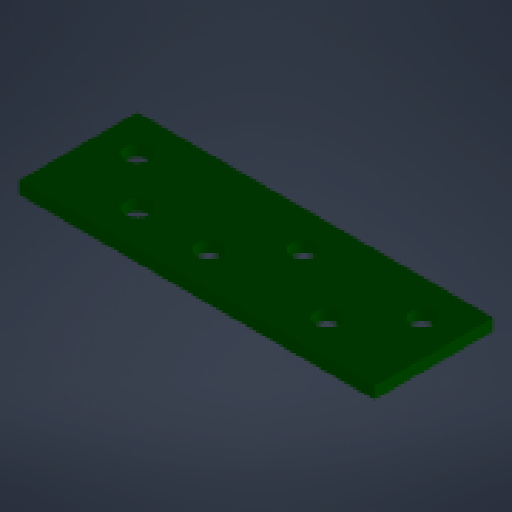
# Autodesk Inventor part: upper_plate
Saved by Autodesk Inventor 2024 (Build 280153000, 153)
## iProperties
Created: 2023-04-16
Part Number: upper_plate
Material: Типовые
Document SubType Name: Modeling
Designer: user
Density: 1 g/cm^3
Appearance: По умолчанию
Author: user
Autodesk Inventor part; units mm, degrees
ref_plane "YZ Plane" through (0, 0, 0) normal (1, 0, 0) x (0, 1, 0)
ref_plane "XZ Plane" through (0, 0, 0) normal (0, 1, 0) x (-1, 0, 0)
ref_plane "XY Plane" through (0, 0, 0) normal (0, 0, 1) x (1, 0, 0)
sketch "Эскиз1" plane through (0, 0, 0) normal (0, 0, 1) x (1, 0, 0)
  line L0 (-10, 0) -> (10, 0) projected
  line L1 (-10, 0) -> (-60, 0) projected
  line L2 (10, -20) -> (60, -20) projected
  circle A0 centre (-16, -14) radius 2 projected
  circle A1 centre (-24, -6) radius 2 projected
  circle A2 centre (-4, -14) radius 2 projected
  circle A3 centre (4, -6) radius 2 projected
  circle A4 centre (16, -14) radius 2 projected
  circle A5 centre (24, -6) radius 2 projected
  line L3 (-30, 0) -> (30, 0)
  line L4 (30, 0) -> (30, -20)
  line L5 (30, -20) -> (-30, -20)
  line L6 (-30, -20) -> (-30, 0)
  point P0 (0, 0)
  point P1 (0, 0)
  dimension "d0" = 60
  constraints: 8 end point, 2 midpoint, 2 parallel, 2 point on line, 1 horizontal, 1 perpendicular
  measures "d0" distance of L3.start L3.end
extrude "Выдавливание1" add sketch "Эскиз1" along normal blind 2
